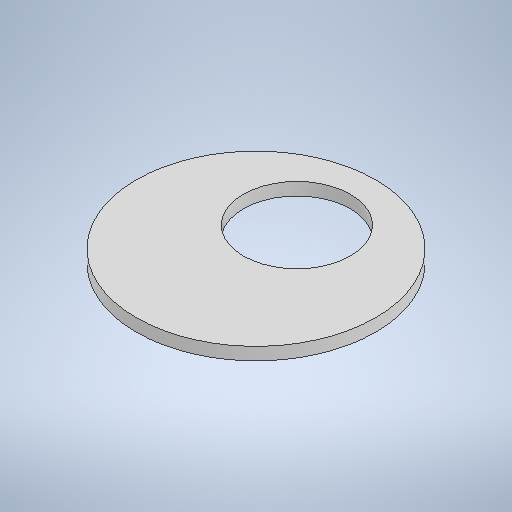
# Autodesk Inventor part: 20.2
Saved by Autodesk Inventor 2025.1 (Build 291241000, 241)
## iProperties
Created: 2024-09-13
Part Number: 20.2
Material: Generisch
Document SubType Name: Modeling
Designer: ffogue
Density: 1 g/cm^3
Appearance: Vorgabe
Author: ffogue
Autodesk Inventor part; units mm, degrees
ref_plane "YZ Plane" through (0, 0, 0) normal (1, 0, 0) x (0, 1, 0)
ref_plane "XZ Plane" through (0, 0, 0) normal (0, 1, 0) x (-1, 0, 0)
ref_plane "XY Plane" through (0, 0, 0) normal (0, 0, 1) x (1, 0, 0)
sketch "Sketch1" plane through (0, 0, 0) normal (0, 0, 1) x (1, 0, 0)
  circle A0 centre (0, 0) radius 9.5
  circle A1 centre (0, 3.25) radius 4.25
  dimension "d0" = 19
  dimension "d1" = 3.25
  dimension "d2" = 8.5
  constraints: 2 centre point, 1 coincident, 1 vertical alignment
  measures "d0" diameter of A0
  measures "d1" distance of point (0, 0) A1.centre
  measures "d2" diameter of A1
extrude "Extrusion1" add sketch "Sketch1" along normal mid plane 1
body "Solid1"
